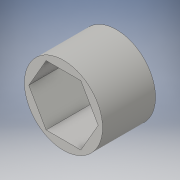
# Autodesk Inventor part: .441Spacer
Saved by Autodesk Inventor 2016 (Build 200138000, 138)
## iProperties
Created: 2016-12-12
Part Number: .441Spacer
Material: Generic
Document SubType Name: Modeling
Designer: Kyle
Density: 1 g/cm^3
Appearance: Default
Mass: 0.707188 g
Surface Area: 10.6181 cm^2
Volume: 0.707188 cm^3
Author: Kyle
Autodesk Inventor part; units mm, degrees
ref_plane "YZ Plane" through (0, 0, 0) normal (1, 0, 0) x (0, 1, 0)
ref_plane "XZ Plane" through (0, 0, 0) normal (0, 1, 0) x (-1, 0, 0)
ref_plane "XY Plane" through (0, 0, 0) normal (0, 0, 1) x (1, 0, 0)
sketch "Sketch2" plane through (0, 0, 0) normal (0, 0, 1) x (1, 0, 0)
  line L0 (0, 12.7) -> (3.6703, 12.7)
  line L1 (0, 12.7) -> (-3.6703, 12.7)
  line L2 (0, 0) -> (3.6703, 0)
  line L3 (0, 0) -> (-3.6703, 0)
  line L4 (-3.6703, 0) -> (-7.3406, 6.35)
  line L5 (-7.3406, 6.35) -> (-3.6703, 12.7)
  line L6 (3.6703, 12.7) -> (7.3406, 6.35)
  line L7 (7.3406, 6.35) -> (3.6703, 0)
  line L8 (0, 0) -> (0, 6.35)
  circle A0 centre (0, 6.35) radius 8.255
  dimension "d11" = 6.35
  dimension "d12" = 16.51
  constraints: 18 end point, 4 horizontal, 1 centre point, 1 coincident, 1 vertical
  measures "d11" distance of L2.start L8.end
  measures "d12" diameter of A0
extrude "Extrusion2" add sketch "Sketch2" along normal blind 6.223
sketch "Sketch3" plane through (0, 6.35, 6.223) normal (0, 0, 1) x (1, 0, 0)
  line L0 (-3.6703, -6.35) -> (-7.3406, 0) projected
  line L1 (-7.3406, 0) -> (-3.6703, 6.35) projected
  line L2 (-3.6703, 6.35) -> (3.6703, 6.35) projected
  line L3 (3.6703, 6.35) -> (7.3406, 0) projected
  line L4 (7.3406, 0) -> (3.6703, -6.35) projected
  line L5 (3.6703, -6.35) -> (-3.6703, -6.35) projected
  circle A0 centre (0, 0) radius 8.255 projected
  point P0 (0, -6.35)
extrude "Extrusion3" add sketch "Sketch3" along normal blind 3.302
sketch "Sketch4" plane through (0, 6.35, 9.525) normal (0, 0, 1) x (1, 0, 0)
  line L0 (-7.3406, 0) -> (-3.6703, 6.35) projected
  line L1 (-3.6703, 6.35) -> (3.6703, 6.35) projected
  line L2 (3.6703, 6.35) -> (7.3406, 0) projected
  line L3 (7.3406, 0) -> (3.6703, -6.35) projected
  line L4 (3.6703, -6.35) -> (-3.6703, -6.35) projected
  line L5 (-3.6703, -6.35) -> (-7.3406, 0) projected
  circle A0 centre (0, 0) radius 8.255 projected
  point P0 (0, -6.35)
extrude "Extrusion4" add sketch "Sketch4" along normal blind 6.5786
sketch "Sketch5" plane through (0, 6.35, 16.1036) normal (0, 0, 1) x (1, 0, 0)
  line L0 (-16.3467, 15.7745) -> (15.1254, 15.7745)
  line L1 (15.1254, 15.7745) -> (15.1254, -12.8793)
  line L2 (15.1254, -12.8793) -> (-16.3467, -12.8793)
  line L3 (-16.3467, -12.8793) -> (-16.3467, 15.7745)
  point P0 (0, -6.35)
  constraints: 8 end point, 2 parallel, 1 horizontal, 1 perpendicular
extrude "Extrusion5" cut sketch "Sketch5" against normal blind 6.5786
sketch "Sketch8" plane through (0, 6.35, 9.525) normal (0, 0, 1) x (1, 0, 0)
  line L0 (-7.3406, 0) -> (-3.6703, -6.35) projected
  line L1 (-3.6703, 6.35) -> (-7.3406, 0) projected
  line L2 (3.6703, 6.35) -> (-3.6703, 6.35) projected
  line L3 (7.3406, 0) -> (3.6703, 6.35) projected
  line L4 (3.6703, -6.35) -> (7.3406, 0) projected
  line L5 (-3.6703, -6.35) -> (3.6703, -6.35) projected
  circle A0 centre (0, 0) radius 8.255 projected
  point P0 (0, -6.35)
extrude "Extrusion7" add sketch "Sketch8" along normal blind 15.875
sketch "Sketch9" plane through (0, 6.35, 25.4) normal (0, 0, 1) x (1, 0, 0)
  line L0 (-7.3406, 0) -> (-3.6703, 6.35) projected
  line L1 (-3.6703, 6.35) -> (3.6703, 6.35) projected
  line L2 (3.6703, 6.35) -> (7.3406, 0) projected
  line L3 (7.3406, 0) -> (3.6703, -6.35) projected
  line L4 (3.6703, -6.35) -> (-3.6703, -6.35) projected
  line L5 (-3.6703, -6.35) -> (-7.3406, 0) projected
  circle A0 centre (0, 0) radius 8.255 projected
  point P0 (0, -6.35)
extrude "Extrusion8" cut sketch "Sketch9" against normal blind 21.7424
sketch "Sketch10" plane through (0, 6.35, 3.6576) normal (0, 0, 1) x (1, 0, 0)
  line L0 (-7.3406, 0) -> (-3.6703, -6.35) projected
  line L1 (-3.6703, 6.35) -> (-7.3406, 0) projected
  line L2 (3.6703, 6.35) -> (-3.6703, 6.35) projected
  line L3 (7.3406, 0) -> (3.6703, 6.35) projected
  line L4 (3.6703, -6.35) -> (7.3406, 0) projected
  line L5 (-3.6703, -6.35) -> (3.6703, -6.35) projected
  circle A0 centre (0, 0) radius 8.255 projected
  point P0 (0, -6.35)
extrude "Extrusion9" add sketch "Sketch10" along normal blind 9.1948
sketch "Sketch11" plane through (0, 6.35, 12.8524) normal (0, 0, 1) x (1, 0, 0)
  line L0 (-15.4934, 11.3446) -> (16.2643, 11.3446)
  line L1 (16.2643, 11.3446) -> (16.2643, -11.0726)
  line L2 (16.2643, -11.0726) -> (-15.4934, -11.0726)
  line L3 (-15.4934, -11.0726) -> (-15.4934, 11.3446)
  point P0 (0, -6.35)
  constraints: 8 end point, 2 parallel, 1 horizontal, 1 perpendicular
extrude "Extrusion10" cut sketch "Sketch11" against normal blind 1.651
body "Solid2"
